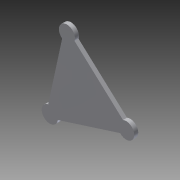
# Autodesk Inventor part: motorPlate
Saved by Autodesk Inventor 2013 (Build 170138000, 138)
## iProperties
Created: 2013-01-08
Part Number: motorPlate
Material: Aluminum 6061
Document SubType Name: Modeling
Designer: Nano
Density: 2.71 g/cm^3
Mass: 168.323 g
Surface Area: 225.935 cm^2
Volume: 62.1116 cm^3
Author: Nano
Autodesk Inventor part; units mm, degrees
ref_plane "YZ Plane" through (0, 0, 0) normal (1, 0, 0) x (0, 1, 0)
ref_plane "XZ Plane" through (0, 0, 0) normal (0, 1, 0) x (-1, 0, 0)
ref_plane "XY Plane" through (0, 0, 0) normal (0, 0, 1) x (1, 0, 0)
sketch "Sketch1" plane through (0, 0, 0) normal (0, 0, 1) x (1, 0, 0)
  circle A0 centre (-32.4028, -72.877) radius 12.7 projected
  circle A1 centre (93.4781, -85.2045) radius 12.7 projected
  circle A2 centre (19.8618, -188.0567) radius 12.7 projected
  line L0 (94.9332, -73.3606) -> (-43.3874, -77.5388)
  line L1 (-43.3874, -77.5388) -> (29.3913, -195.2388)
  line L2 (29.3913, -195.2388) -> (94.9332, -73.3606)
  point P0 (0, 0)
  point P1 (-39.9576, -83.0855)
  point P2 (-20.3377, -76.8425)
  point P3 (88.4146, -73.5575)
  point P4 (84.0113, -93.6703)
  point P5 (17.2635, -175.6253)
  point P6 (32.48, -189.4951)
  constraints: 6 end point, 6 point on circle, 6 point on line
extrude "Extrusion1" add sketch "Sketch1" along normal blind 6.35
body "Solid1"
